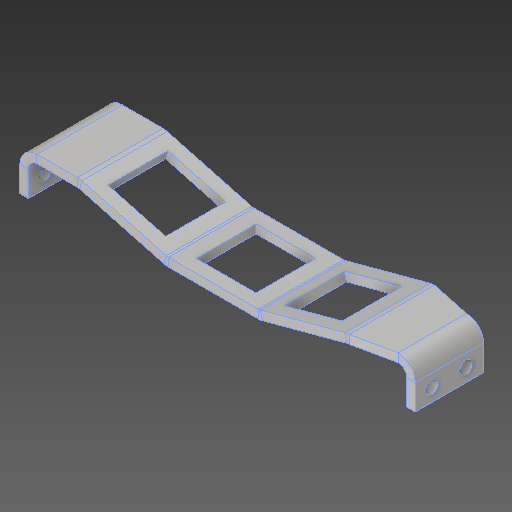
# Autodesk Inventor part: keyplate3
Saved by Autodesk Inventor 2018 (Build 220112000, 112)
## iProperties
Created: 2018-05-25
Part Number: keyplate3
Material: アルミニウム 6061
Document SubType Name: Sheet Metal
Designer: NaMACHAN
Density: 2.7 g/cm^3
Sheet Metal Rule: Al2mm
Appearance: アルミニウム - フラット
Mass: 7.72809 g
Surface Area: 37.6833 cm^2
Volume: 2.86226 cm^3
Author: NaMACHAN
Autodesk Inventor part; units mm, degrees
ref_plane "YZ Plane" through (0, 0, 0) normal (1, 0, 0) x (0, 1, 0)
ref_plane "XZ Plane" through (0, 0, 0) normal (0, 1, 0) x (-1, 0, 0)
ref_plane "XY Plane" through (0, 0, 0) normal (0, 0, 1) x (1, 0, 0)
sketch "スケッチ1" plane through (0, 0, 0) normal (0, 1, 0) x (-1, 0, 0)
  line L0 (-10.5, -10) -> (10.5, -10)
  line L1 (10.5, -10) -> (10.5, 10)
  line L2 (10.5, 10) -> (-10.5, 10)
  line L3 (-10.5, 10) -> (-10.5, -10)
  line L4 (-10.5, -10) -> (10.5, 10) construction
  line L5 (10.5, -10) -> (-10.5, 10) construction
  line L6 (-7, -7) -> (7, -7)
  line L7 (7, -7) -> (7, 7)
  line L8 (7, 7) -> (-7, 7)
  line L9 (-7, 7) -> (-7, -7)
  line L10 (-7, -7) -> (7, 7) construction
  line L11 (7, -7) -> (-7, 7) construction
  point P0 (0, 0)
  dimension "d0" = 21
  dimension "d1" = 20
  dimension "d2" = 14
  dimension "d3" = 14
  measures "d0" distance of L2.end L1.end
  measures "d1" distance of L1.end L0.end
  measures "d2" distance of L8.end L7.end
  measures "d3" distance of L7.end L6.end
extrude "プレート1" add sketch "スケッチ1" along normal blind 2
sketch "スケッチ2" plane through (-11.0176, 2.0681, 10) normal (-0.258819, -0.9659258, 0) x (0.9659258, -0.258819, 0)
  line L0 (0, -20) -> (0, 0)
  line L1 (0, 0) -> (-20.4734, 0)
  line L2 (-20.4734, 0) -> (-20.4734, -20)
  line L3 (-20.4734, -20) -> (0, -20)
  constraints: 6 end point, 1 horizontal, 1 perpendicular, 1 vertical
edge flange "フランジ1" height 21 angle 15 thickness 2 bend radius 2 thickness toward (-0.258819, -0.9659258, 0) relief straight relief width 2 relief depth 1 edges at (-10.5, 2, 0) wall of the first edge with corners at (-11.0176, 2.0681, -10) (-11.0176, 2.0681, 10) (-30.7934, 7.3671, 10) (-30.7934, 7.3671, -10)
bend "曲げ1"
corner "コーナー1"
sketch "スケッチ3" plane through (11.0176, 2.0681, -10) normal (0.258819, -0.9659258, 0) x (0.9659258, 0.258819, 0)
  line L0 (0, 20) -> (0, 0)
  line L1 (0, 0) -> (20.4734, 0)
  line L2 (20.4734, 0) -> (20.4734, 20)
  line L3 (20.4734, 20) -> (0, 20)
  constraints: 8 end point
edge flange "フランジ2" height 21 angle 15 thickness 2 bend radius 2 thickness toward (0.258819, -0.9659258, 0) relief straight relief width 2 relief depth 1 edges at (10.5, 2, 0) wall of the first edge with corners at (11.0176, 2.0681, 10) (11.0176, 2.0681, -10) (30.7934, 7.3671, -10) (30.7934, 7.3671, 10)
bend "曲げ2"
corner "コーナー2"
sketch "スケッチ6" plane through (-31.8287, 5.5033, 10) normal (0, 1, 0) x (1, 0, 0)
  line L0 (0, -20) -> (0, 0)
  line L1 (0, 0) -> (-9.4734, 0)
  line L2 (-9.4734, 0) -> (-9.4734, -20)
  line L3 (-9.4734, -20) -> (0, -20)
  constraints: 8 end point
edge flange "フランジ5" height 10 angle -15 thickness 2 bend radius 2 thickness toward (0, 1, 0) relief straight relief width 2 relief depth 1 edges at (-30.7934, 7.3671, 0) wall of the first edge with corners at (-31.8287, 5.5033, -10) (-31.8287, 5.5033, 10) (-41.3021, 5.5033, 10) (-41.3021, 5.5033, -10)
bend "曲げ5"
corner "コーナー5"
sketch "スケッチ7" plane through (11.0176, 2.0681, 10) normal (-0.258819, 0.9659258, 0) x (0.9659258, 0.258819, 0)
  line L0 (2.7367, 17) -> (16.7367, 17)
  line L1 (16.7367, 17) -> (16.7367, 3)
  line L2 (16.7367, 3) -> (2.7367, 3)
  line L3 (2.7367, 3) -> (2.7367, 17)
  line L4 (2.7367, 17) -> (16.7367, 3) construction
  line L5 (16.7367, 17) -> (2.7367, 3) construction
  line L6 (20.4734, 0) -> (0, 0) projected
  line L7 (-0.5176, 20) -> (-0.5176, 0) projected
  point P0 (-11.1775, 10)
  point P1 (9.7367, 10)
  point P2 (9.7367, 10)
  point P3 (9.7367, 0)
  point P4 (19.4734, 0)
  point P5 (9.7367, 10)
  point P6 (-0.5176, 10)
  dimension "d55" = 14
  dimension "d56" = 14
  constraints: 12 end point, 5 midpoint, 2 parallel, 1 horizontal, 1 horizontal alignment, 1 perpendicular, 1 point on line, 1 vertical alignment
  measures "d55" distance of L1.end L2.end
  measures "d56" distance of L0.end L1.end
extrude "押し出し1" cut sketch "スケッチ7" against normal blind 10
sketch "スケッチ9" plane through (-11.0176, 2.0681, 10) normal (0.258819, 0.9659258, 0) x (0.9659258, -0.258819, 0)
  line L0 (-17.2367, 17) -> (-3.2367, 17)
  line L1 (-3.2367, 17) -> (-3.2367, 3)
  line L2 (-3.2367, 3) -> (-17.2367, 3)
  line L3 (-17.2367, 3) -> (-17.2367, 17)
  line L4 (-17.2367, 17) -> (-3.2367, 3) construction
  line L5 (-3.2367, 17) -> (-17.2367, 3) construction
  line L6 (-20.4734, 20) -> (-20.4734, 0) projected
  line L7 (-20.4734, 0) -> (0, 0) projected
  point P0 (11.1775, 10)
  point P1 (-10.2367, 10)
  point P2 (-10.2367, 10)
  point P3 (-20.4734, 10)
  point P4 (-10.2367, 10)
  point P5 (-10.2367, 0)
  dimension "d63" = 14
  dimension "d64" = 14
  constraints: 12 end point, 6 midpoint, 2 parallel, 1 horizontal, 1 horizontal alignment, 1 perpendicular, 1 vertical alignment
  measures "d63" distance of L1.end L2.end
  measures "d64" distance of L0.end L1.end
extrude "押し出し3" cut sketch "スケッチ9" against normal blind 10
sketch "スケッチ14" plane through (31.8287, 5.5033, -10) normal (0, 1, 0) x (1, 0, 0)
  line L0 (0, 20) -> (0, 0)
  line L1 (0, 0) -> (9.4734, 0)
  line L2 (9.4734, 0) -> (9.4734, 20)
  line L3 (9.4734, 20) -> (0, 20)
  constraints: 6 end point, 1 horizontal, 1 perpendicular, 1 vertical
edge flange "フランジ6" height 10 angle -15 thickness 2 bend radius 2 thickness toward (0, 1, 0) relief straight relief width 2 relief depth 1 edges at (30.7934, 7.3671, 0) wall of the first edge with corners at (31.8287, 5.5033, 10) (31.8287, 5.5033, -10) (41.3021, 5.5033, -10) (41.3021, 5.5033, 10)
bend "曲げ6"
corner "コーナー6"
sketch "スケッチ20" plane through (41.3021, 7.5033, 10) normal (0, 1, 0) x (1, 0, 0)
  line L0 (0, 0) -> (0, 20) projected
  line L1 (0, 20) -> (0, 18)
  line L2 (0, 20) -> (-9.4734, 20) projected
  line L3 (0, 18) -> (-9.4734, 20)
  line L4 (-9.4734, 0) -> (0, 0) projected
  line L5 (-9.4734, 0) -> (0, 0)
  line L6 (0, 0) -> (0, 2)
  line L7 (-9.4734, 0) -> (0, 2)
  line L8 (-9.4734, 20) -> (0, 20)
  point P0 (-41.3021, 10)
  dimension "d150" = 2
  dimension "d151" = 2
  constraints: 12 end point, 2 collinear, 2 point on line, 1 perpendicular
  measures "d150" distance of L0.end L1.end
  measures "d151" distance of L0.start L6.end
extrude "押し出し9" cut sketch "スケッチ20" against normal blind 10
sketch "スケッチ22" plane through (43.3021, 3.5033, 8) normal (1, 0, 0) x (0, 1, 0)
  line L0 (0, -16) -> (0, 0)
  line L1 (0, 0) -> (-6, 0)
  line L2 (-6, 0) -> (-6, -16)
  line L3 (-6, -16) -> (0, -16)
  constraints: 6 end point, 1 horizontal, 1 perpendicular, 1 vertical
edge flange "フランジ11" height 10 angle 90 thickness 2 bend radius 2 thickness toward (1, 0, 0) relief straight relief width 2 relief depth 1 edges at (41.3021, 5.5033, 0) wall of the first edge with corners at (43.3021, 3.5033, -8) (43.3021, 3.5033, 8) (43.3021, -2.4967, 8) (43.3021, -2.4967, -8)
bend "曲げ11"
corner "コーナー11"
sketch "スケッチ23" plane through (-43.3021, 3.5033, -10) normal (-1, 0, 0) x (0, -1, 0)
  line L0 (0, 20) -> (0, 0)
  line L1 (0, 0) -> (6, 0)
  line L2 (6, 0) -> (6, 20)
  line L3 (6, 20) -> (0, 20)
  constraints: 6 end point, 1 horizontal, 1 perpendicular, 1 vertical
edge flange "フランジ12" height 10 angle 90 thickness 2 bend radius 2 thickness toward (-1, 0, 0) relief straight relief width 2 relief depth 1 edges at (-41.3021, 5.5033, 0) wall of the first edge with corners at (-43.3021, 3.5033, 10) (-43.3021, 3.5033, -10) (-43.3021, -2.4967, -10) (-43.3021, -2.4967, 10)
bend "曲げ12"
corner "コーナー12"
sketch "スケッチ24" plane through (45.3021, -2.4967, 8) normal (1, 0, 0) x (0, 0, -1)
  line L0 (16, 6) -> (16, 0) projected
  line L1 (0, 0) -> (0, 6) projected
  point P0 (8, 2.4967)
  point P1 (4, 3)
  point P2 (12, 3)
  point P3 (16, 3)
  dimension "d185" = 4
  dimension "d186" = 4
  constraints: 2 horizontal alignment, 1 midpoint
  measures "d185" distance from line of point (12, 3) L0
  measures "d186" distance from line of L1 point (4, 3)
hole "穴2" at (45.3021, 0.5033, 4) at (45.3021, 0.5033, -4) direction (-1, 0, 0) diameter 3 depth 2 tip angle 118
sketch "スケッチ25" plane through (-45.3021, -2.4967, -10) normal (-1, 0, 0) x (0, 0, 1)
  line L0 (0, 0) -> (0, 6) projected
  line L1 (20, 6) -> (20, 0) projected
  point P0 (10, 2.4967)
  point P1 (4, 3)
  point P2 (16, 3)
  point P3 (0, 3)
  dimension "d194" = 4
  dimension "d195" = 4
  constraints: 2 horizontal alignment, 1 midpoint
  measures "d194" distance from line of L0 point (4, 3)
  measures "d195" distance from line of L1 point (16, 3)
hole "穴3" at (-45.3021, 0.5033, -6) at (-45.3021, 0.5033, 6) direction (1, 0, 0) diameter 3 depth 2 tip angle 118
equation "\"d192\" = Thickness"
equation "\"d201\" = Thickness"
equation "\"d4\" = Thickness"
equation "\"d5\" = BendReliefWidth"
equation "\"d6\" = BendReliefDepth"
equation "\"d7\" = MinimumRemnant"
equation "\"d8\" = TransitionRadius"
equation "\"d11\" = BendRadius"
equation "\"d12\" = CornerReliefSize"
equation "\"d13\" = GapSize"
equation "\"d14\" = JacobiRadiusSize"
equation "\"d15\" = BendReliefWidth"
equation "\"d16\" = BendReliefDepth"
equation "\"d17\" = MinimumRemnant"
equation "\"d18\" = TransitionRadius"
equation "\"d21\" = BendRadius"
equation "\"d22\" = CornerReliefSize"
equation "\"d23\" = GapSize"
equation "\"d24\" = JacobiRadiusSize"
equation "\"d45\" = BendReliefWidth"
equation "\"d46\" = BendReliefDepth"
equation "\"d47\" = MinimumRemnant"
equation "\"d48\" = TransitionRadius"
equation "\"d51\" = BendRadius"
equation "\"d52\" = CornerReliefSize"
equation "\"d53\" = GapSize"
equation "\"d54\" = JacobiRadiusSize"
equation "\"d83\" = BendReliefWidth"
equation "\"d84\" = BendReliefDepth"
equation "\"d85\" = MinimumRemnant"
equation "\"d86\" = TransitionRadius"
equation "\"d89\" = BendRadius"
equation "\"d90\" = CornerReliefSize"
equation "\"d91\" = GapSize"
equation "\"d92\" = JacobiRadiusSize"
equation "\"d165\" = BendReliefWidth"
equation "\"d166\" = BendReliefDepth"
equation "\"d167\" = MinimumRemnant"
equation "\"d168\" = TransitionRadius"
equation "\"d171\" = BendRadius"
equation "\"d172\" = CornerReliefSize"
equation "\"d173\" = GapSize"
equation "\"d174\" = JacobiRadiusSize"
equation "\"d175\" = BendReliefWidth"
equation "\"d176\" = BendReliefDepth"
equation "\"d177\" = MinimumRemnant"
equation "\"d178\" = TransitionRadius"
equation "\"d181\" = BendRadius"
equation "\"d182\" = CornerReliefSize"
equation "\"d183\" = GapSize"
equation "\"d184\" = JacobiRadiusSize"
equation "\"BendRadius\" = Thickness"
equation "\"BendReliefWidth\" = Thickness"
equation "\"BendReliefDepth\" = 0.5 * Thickness"
equation "\"CornerReliefSize\" = 4 * Thickness"
equation "\"MinimumRemnant\" = 2 * Thickness"
equation "\"TransitionRadius\" = BendRadius"
equation "\"JacobiRadiusSize\" = BendRadius"
equation "\"GapSize\" = Thickness"
equation "\"Thickness\" = 2"
